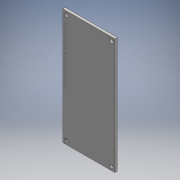
# Autodesk Inventor part: PCB
Saved by Autodesk Inventor 2016 (Build 200138000, 138)
## iProperties
Created: 2016-04-16
Part Number: PCB
Material: Generic
Document SubType Name: Modeling
Designer: Jarrett
Density: 1 g/cm^3
Appearance: Default
Author: Jarrett
Autodesk Inventor part; units mm, degrees
ref_plane "YZ Plane" through (0, 0, 0) normal (1, 0, 0) x (0, 1, 0)
ref_plane "XZ Plane" through (0, 0, 0) normal (0, 1, 0) x (-1, 0, 0)
ref_plane "XY Plane" through (0, 0, 0) normal (0, 0, 1) x (1, 0, 0)
sketch "Sketch1" plane through (0, 0, 0) normal (0, 1, 0) x (-1, 0, 0)
  line L0 (0, 0) -> (36, 0)
  line L1 (36, 0) -> (36, -80)
  line L2 (36, -80) -> (0, -80)
  line L3 (0, -80) -> (0, 0)
  dimension "d0" = 80
  dimension "d1" = 36
  constraints: 8 end point, 2 parallel, 1 horizontal, 1 perpendicular
  measures "d0" distance of L0.end L1.end
  measures "d1" distance of L0.start L0.end
extrude "Extrusion1" add sketch "Sketch1" along normal blind 1.6
sketch "Sketch2" plane through (0, 1.6, 0) normal (0, 1, 0) x (1, 0, 0)
  line L0 (-36, 80) -> (-36, 0) projected
  line L1 (-36, 2.5) -> (0, 2.5) construction
  line L2 (0, 0) -> (0, 80) projected
  line L3 (-36, 77.5) -> (0, 77.5) construction
  line L4 (-33.5, 47.8636) -> (-33.5, 0) construction
  line L5 (-36, 0) -> (0, 0) projected
  line L6 (-2.5, 0) -> (-2.5, 80) construction
  line L7 (0, 80) -> (-36, 80) projected
  circle A0 centre (-33.5, 2.5) radius 1.25
  circle A1 centre (-2.5, 2.5) radius 1.25
  circle A2 centre (-33.5, 77.5) radius 1.25
  circle A3 centre (-2.5, 77.5) radius 1.25
  dimension "d4" = 2.5
  dimension "d5" = 2.5
  dimension "d6" = 2.5
  dimension "d7" = 2.5
  dimension "d8" = 2.5
  constraints: 15 point on line, 8 end point, 4 centre point, 3 equal radius, 3 perpendicular, 1 horizontal
  measures "d4" diameter of A0
  measures "d5" distance between parallel lines of L5 L1
  measures "d6" distance between parallel lines of L0 L4
  measures "d7" distance between parallel lines of L2 L6
  measures "d8" distance between parallel lines of L7 L3
extrude "Extrusion2" cut sketch "Sketch2" against normal up to next contours A0 | A1 | A2 | A3
sketch "Sketch3" plane through (0, 1.6, 0) normal (0, 1, 0) x (1, 0, 0)
  line L0 (0, 0) -> (-36, 0) projected
  line L1 (-34, 0) -> (-34, 80) construction
  line L2 (-36, 80) -> (0, 80) projected
  line L3 (-36, 80) -> (-36, 0) projected
  circle A0 centre (-34, 8) radius 0.5
  circle A1 centre (-34, 10.5) radius 0.5
  circle A2 centre (-34, 13) radius 0.5
  circle A3 centre (-34, 15.5) radius 0.5
  circle A4 centre (-34, 18) radius 0.5
  circle A5 centre (-34, 20.5) radius 0.5
  circle A6 centre (-34, 23) radius 0.5
  circle A7 centre (-34, 25.5) radius 0.5
  circle A8 centre (-34, 28) radius 0.5
  circle A9 centre (-34, 30.5) radius 0.5
  circle A10 centre (-34, 33) radius 0.5
  circle A11 centre (-34, 35.5) radius 0.5
  circle A12 centre (-34, 38) radius 0.5
  circle A13 centre (-34, 40.5) radius 0.5
  circle A14 centre (-34, 43) radius 0.5
  circle A15 centre (-34, 45.5) radius 0.5
  dimension "d11" = 2
  dimension "d12" = 1
  dimension "d13" = 8
  dimension "d16" = 2.5
  constraints: 16 centre point, 3 point on line, 2 end point, 1 perpendicular, 1 vertical, 30 other
  measures "d11" distance between parallel lines of L1 L3
  measures "d12" diameter of A0
  measures "d13" distance from line of L0 A0.centre
  measures "d16" distance of A0.centre A1.centre
extrude "Extrusion3" cut sketch "Sketch3" against normal up to next
body "Solid1"
